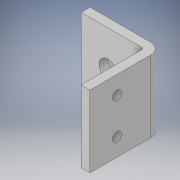
# Autodesk Inventor part: Soporte
Saved by Autodesk Inventor 2019 (Build 230136000, 136)
## iProperties
Created: 2019-05-14
Part Number: Soporte
Material: Generic
Document SubType Name: Modeling
Designer: Gustavo Marin
Density: 1 g/cm^3
Appearance: Default
Author: Gustavo Marin
Autodesk Inventor part; units mm, degrees
ref_plane "YZ Plane" through (0, 0, 0) normal (1, 0, 0) x (0, 1, 0)
ref_plane "XZ Plane" through (0, 0, 0) normal (0, 1, 0) x (-1, 0, 0)
ref_plane "XY Plane" through (0, 0, 0) normal (0, 0, 1) x (1, 0, 0)
sketch "Sketch1" plane through (0, 0, 0) normal (0, 1, 0) x (-1, 0, 0)
  line L0 (0, 0) -> (0, -85.725)
  line L1 (15.875, -101.6) -> (101.6, -101.6)
  line L2 (101.6, -101.6) -> (101.6, -88.9)
  line L3 (101.6, -88.9) -> (12.7, -88.9)
  line L4 (12.7, -88.9) -> (12.7, 0)
  line L5 (12.7, 0) -> (0, 0)
  arc A0 (0, -85.725) -> (15.875, -101.6) centre (15.875, -85.725) ccw
  arc A1 (0, -85.725) -> (15.875, -101.6) centre (15.875, -85.725) ccw
  point P0 (0, -101.6)
  dimension "d0" = 101.6
  dimension "d1" = 101.6
  dimension "d2" = 12.7
  dimension "d3" = 12.7
  dimension "d4" = 15.875
  dimension "d5" = 15.875
  constraints: 12 end point, 5 perpendicular, 4 point on circle, 4 point on line, 4 tangent, 2 centre point, 1 vertical
  measures "d0" distance of L0.start point (0, -101.6)
  measures "d1" distance of point (0, -101.6) L1.end
  measures "d2" distance between parallel lines of L4 L0
  measures "d3" distance between parallel lines of L3 L1
  measures "d4" radius of A0
  measures "d5" radius of A1
extrude "Extrusion1" add sketch "Sketch1" along normal blind 101.6
sketch "Sketch2" plane through (-12.7, 0, -88.9) normal (-1, 0, 0) x (0, 0, 1)
  circle A0 centre (50.8, 25.4) radius 6.35
  circle A1 centre (50.8, 76.2) radius 6.35
  line L0 (0, 0) -> (88.9, 0) projected
  line L1 (88.9, 0) -> (88.9, 101.6) projected
  dimension "d8" = 12.7
  dimension "d9" = 12.7
  dimension "d10" = 25.4
  dimension "d11" = 50.8
  dimension "d12" = 38.1
  dimension "d13" = 38.1
  constraints: 2 centre point
  measures "d8" diameter of A0
  measures "d9" diameter of A1
  measures "d10" distance from line of L0 A0.centre
  measures "d11" distance of A0.centre A1.centre
  measures "d12" distance from line of L1 A0.centre
  measures "d13" distance from line of L1 A1.centre
extrude "Extrusion2" cut sketch "Sketch2" against normal blind 101.6
sketch "Sketch3" plane through (-101.6, 0, -88.9) normal (0, 0, 1) x (1, 0, 0)
  circle A0 centre (38.1, 50.8) radius 12.7
  line L0 (0, 0) -> (0, 101.6) projected
  line L1 (0, 101.6) -> (88.9, 101.6) projected
  point P0 (101.6, 0)
  dimension "d16" = 25.4
  dimension "d17" = 38.1
  dimension "d18" = 50.8
  constraints: 1 centre point
  measures "d16" diameter of A0
  measures "d17" distance from line of L0 A0.centre
  measures "d18" distance from line of L1 A0.centre
extrude "Extrusion3" cut sketch "Sketch3" against normal blind 101.6
fillet "Fillet1" radius 3.175 1 edges at (-12.7, 50.8, -88.9)
body "Solid1"
